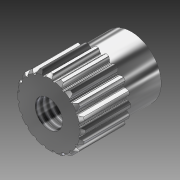
# Autodesk Inventor part: Tower Pro Servo Spline Shaft End
Saved by Autodesk Inventor 2013 SP2 (Build 170200200, 200)
## iProperties
Created: 2020-02-23
Part Number: Tower Pro Servo Spline Shaft End
Material: Generic
Document SubType Name: Modeling
Designer: DELL
Density: 1 g/cm^3
Author: DELL
Autodesk Inventor part; units mm, degrees
ref_plane "YZ Plane" through (0, 0, 0) normal (1, 0, 0) x (0, 1, 0)
ref_plane "XZ Plane" through (0, 0, 0) normal (0, 1, 0) x (-1, 0, 0)
ref_plane "XY Plane" through (0, 0, 0) normal (0, 0, 1) x (1, 0, 0)
sketch "Sketch1" plane through (0, 0, 0) normal (0, 0, 1) x (1, 0, 0)
  arc A0 (0.2576, 2.2013) -> (0.3072, 2.1617) centre (0.3159, 2.2235) ccw
  arc A1 (0.2576, 2.2013) -> (0.2432, 2.2368) centre (-0.6912, 1.8391) ccw
  spline S0 degree 3 poles (0.2432, 2.2368) (0.2078, 2.32) (0.1605, 2.3999) (0.1023, 2.4729) knots 0.326859 0.326859 0.326859 0.326859 0.361037 0.361037 0.361037 0.361037 construction
  arc A2 (0.1023, 2.4729) -> (-0.1023, 2.4729) centre (0, 0) ccw construction
  spline S1 degree 3 poles (-0.1023, 2.4729) (-0.1605, 2.3999) (-0.2078, 2.32) (-0.2432, 2.2368) knots 0.628056 0.628056 0.628056 0.628056 0.662234 0.662234 0.662234 0.662234 construction
  arc A3 (-0.2432, 2.2368) -> (-0.2576, 2.2013) centre (0.6912, 1.8391) ccw
  arc A4 (-0.3072, 2.1617) -> (-0.2576, 2.2013) centre (-0.3159, 2.2235) ccw
  line L0 (0, -3.1161) -> (0, 3.4128) construction
  circle A5 centre (0, 0) radius 2.1834
  point P0 (0, 0)
  point P1 (0, 0)
  dimension "d12" = 4.3668
  dimension "d0" = 2.475
  dimension "d1" = 2.2235
  dimension "d2" = 0.6912
  dimension "d3" = 1.3823
  dimension "d4" = 1.8391
  dimension "d5" = 0.316
  dimension "d6" = 0.6319
  dimension "d7" = 0.0625
  dimension "d8" = 1.0155
  constraints: 10 point on circle, 5 centre point, 3 coincident, 2 horizontal alignment, 1 equal radius, 9 other
  measures "d0" radius of A2
  measures "d1" vertical distance of A0.centre point (0, 0)
  measures "d2" distance from line of A3.centre L0
  measures "d3" distance of A3.centre A1.centre
  measures "d4" vertical distance of A3.centre point (0, 0)
  measures "d5" distance from line of A0.centre L0
  measures "d6" distance of A0.centre A4.centre
  measures "d7" radius of A0
  measures "d8" radius of A3
extrude "Extrusion1" add sketch "Sketch1" against normal blind 6
sketch "Sketch2" plane through (0, 0, 0) normal (0, 0, 1) x (1, 0, 0)
  arc A0 (0.1023, 2.4729) -> (-0.1023, 2.4729) centre (0, 0) ccw projected
  spline S0 degree 3 poles (0.2432, 2.2368) (0.2078, 2.32) (0.1605, 2.3999) (0.1023, 2.4729) knots 0.326859 0.326859 0.326859 0.326859 0.361037 0.361037 0.361037 0.361037 projected
  spline S1 degree 3 poles (-0.1023, 2.4729) (-0.1605, 2.3999) (-0.2078, 2.32) (-0.2432, 2.2368) knots 0.628056 0.628056 0.628056 0.628056 0.662234 0.662234 0.662234 0.662234 projected
  arc A1 (-0.2432, 2.2368) -> (-0.2576, 2.2013) centre (0.6912, 1.8391) ccw projected
  arc A2 (-0.3072, 2.1617) -> (-0.2576, 2.2013) centre (-0.3159, 2.2235) ccw projected
  arc A3 (0.2576, 2.2013) -> (0.2432, 2.2368) centre (-0.6912, 1.8391) ccw projected
  arc A4 (0.2576, 2.2013) -> (0.3072, 2.1617) centre (0.3159, 2.2235) ccw projected
  arc A5 (0.3072, 2.1617) -> (-0.3072, 2.1617) centre (0, 0) ccw
  point P0 (0, 0)
  dimension "d15" = 2.1834
  constraints: 4 point on circle, 1 centre point
  measures "d15" radius of A5
extrude "Extrusion2" add sketch "Sketch2" against normal blind 3.5
pattern_circular "Circular Pattern1" count 20 over 360 about axis through (0, 0, 0) along (0, 0, -1) of "Extrusion2"
sketch "Sketch3" plane through (0, 0, 0) normal (0, 0, 1) x (1, 0, 0)
  point P0 (0, 0)
chamfer "Chamfer1" distance 0.2 angle 45 20 edges at (1.4548, 2.0023, 0) (2.0023, 1.4548, 0) (2.3539, 0.7648, 0) (2.475, 0, 0) (2.3539, -0.7648, 0) (2.0023, -1.4548, 0) (1.4548, -2.0023, 0) (0.7648, -2.3539, 0) (0, -2.475, 0) (-0.7648, -2.3539, 0) (-1.4548, -2.0023, 0) (-2.0023, -1.4548, 0) (-2.3539, -0.7648, 0) (-2.475, 0, 0) (-2.3539, 0.7648, 0) (-2.0023, 1.4548, 0) (-1.4548, 2.0023, 0) (-0.7648, 2.3539, 0) (0, 2.475, 0) (0.7648, 2.3539, 0)
sketch "Sketch4" plane through (0, 0, 0) normal (0, 0, 1) x (1, 0, 0)
  point P0 (0, 0)
hole "Hole1" at (0, 0, 0) direction (0, 0, -1) diameter 2.013 depth 5 thread size "M2.5x0.45" class "6H" standard "ANSI Metric M Profile"
body "Solid1"
